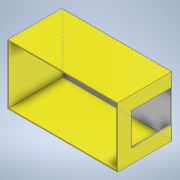
# Autodesk Inventor part: Room_0RC039
Saved by Autodesk Inventor 2022 (Build 260153000, 153)
## iProperties
Created: 2021-06-29
Part Number: Room_0RC039
Material: Generic
Document SubType Name: Modeling
Designer: jamieson-bl
Density: 1 g/cm^3
Appearance: Default
Author: jamieson-bl
Autodesk Inventor part; units mm, degrees
ref_plane "YZ Plane" through (0, 0, 0) normal (1, 0, 0) x (0, 1, 0)
ref_plane "XZ Plane" through (0, 0, 0) normal (0, 1, 0) x (-1, 0, 0)
ref_plane "XY Plane" through (0, 0, 0) normal (0, 0, 1) x (1, 0, 0)
sketch "Sketch1" plane through (0, 0, 0) normal (0, 0, 1) x (1, 0, 0)
  line L0 (2726.5313, -1465.2625) -> (-2726.5312, -1465.2625)
  line L1 (-2726.5312, -1465.2625) -> (-2726.5312, 1465.2625)
  line L2 (-2726.5312, 1465.2625) -> (2726.5313, 1465.2625)
  line L3 (2726.5313, 1465.2625) -> (2726.5313, -1465.2625)
  line L4 (2726.5313, -1465.2625) -> (-2726.5312, 1465.2625) construction
  line L5 (-2726.5312, -1465.2625) -> (2726.5313, 1465.2625) construction
  point P0 (0, 0)
  dimension "d0" = 5453.0625
  dimension "d1" = 2930.525
  constraints: 12 end point, 2 midpoint, 2 parallel, 1 horizontal, 1 perpendicular
  measures "d0" distance of L1.end L2.end
  measures "d1" distance of L0.end L1.end
extrude "Extrusion1" add sketch "Sketch1" along normal blind 25.4
sketch "Sketch2" plane through (0, 0, 25.4) normal (0, 0, 1) x (1, 0, 0)
  line L0 (2726.5313, 1465.2625) -> (-2726.5312, 1465.2625) projected
  line L1 (2726.5312, -1465.2625) -> (-2726.5312, -1465.2625)
  line L2 (-2726.5312, -1465.2625) -> (-2726.5312, 1465.2625)
  line L3 (-2726.5312, 1465.2625) -> (2726.5312, 1465.2625)
  line L4 (2726.5312, 1465.2625) -> (2726.5312, -1465.2625)
  line L5 (2726.5312, -1465.2625) -> (-2726.5312, 1465.2625) construction
  line L6 (-2726.5312, -1465.2625) -> (2726.5312, 1465.2625) construction
  line L7 (2777.3376, -1516.0625) -> (-2777.3376, -1516.0625)
  line L8 (-2777.3376, -1516.0625) -> (-2777.3376, 1516.0625)
  line L9 (-2777.3376, 1516.0625) -> (2777.3376, 1516.0625)
  line L10 (2777.3376, 1516.0625) -> (2777.3376, -1516.0625)
  line L11 (2777.3376, -1516.0625) -> (-2777.3376, 1516.0625) construction
  line L12 (-2777.3376, -1516.0625) -> (2777.3376, 1516.0625) construction
  point P0 (0, 0)
  dimension "d4" = 5554.6752
  dimension "d5" = 3032.125
  constraints: 24 end point, 4 midpoint, 4 parallel, 2 horizontal, 2 perpendicular
  measures "d4" distance of L8.end L9.end
  measures "d5" distance of L7.end L8.end
extrude "Extrusion2" add sketch "Sketch2" along normal blind 2743.2
sketch "Sketch3" plane through (2777.3376, -1516.0625, 25.4) normal (1, 0, 0) x (0, 0, -1)
  line L0 (0, 50.8) -> (0, 2981.325) projected
  line L1 (0, 711.2) -> (-2032, 711.2)
  line L2 (-2032, 711.2) -> (-2032, 2336.8)
  line L3 (-2032, 2336.8) -> (0, 2336.8)
  line L4 (0, 2336.8) -> (0, 711.2)
  point P0 (25.4, 1516.0625)
  point P1 (0, 2336.8)
  dimension "d8" = 2032
  dimension "d9" = 1625.6
  constraints: 8 end point, 2 parallel, 1 horizontal, 1 perpendicular, 1 point on line
  measures "d8" distance of L2.end L3.end
  measures "d9" distance of L1.end L2.end
extrude "Extrusion3" cut sketch "Sketch3" against normal up to next
body "Solid1"
